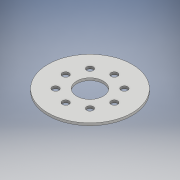
# Autodesk Inventor part: motor_spacer_leg
Saved by Autodesk Inventor 2018 (Build 220112000, 112)
## iProperties
Created: 2018-05-21
Part Number: motor_spacer_leg
Material: Generic
Document SubType Name: Modeling
Designer: bitbots
Density: 1 g/cm^3
Appearance: Default
Author: bitbots
Autodesk Inventor part; units mm, degrees
ref_plane "YZ Plane" through (0, 0, 0) normal (1, 0, 0) x (0, 1, 0)
ref_plane "XZ Plane" through (0, 0, 0) normal (0, 1, 0) x (-1, 0, 0)
ref_plane "XY Plane" through (0, 0, 0) normal (0, 0, 1) x (1, 0, 0)
sketch "Sketch1" plane through (0, 0, 0) normal (0, 0, 1) x (1, 0, 0)
  line L0 (-13, -11) -> (13, -11) construction
  circle A0 centre (0, 0) radius 13.8 construction
  circle A1 centre (0, 0) radius 5 construction
  circle A2 centre (0, -11) radius 1.2813 construction
  circle A3 centre (-7.7782, -7.7782) radius 1.2813 construction
  circle A4 centre (-11, 0) radius 1.2813 construction
  circle A5 centre (-7.7782, 7.7782) radius 1.2813 construction
  circle A6 centre (0, 11) radius 1.2813 construction
  circle A7 centre (7.7782, 7.7782) radius 1.2813 construction
  circle A8 centre (11, 0) radius 1.2813 construction
  circle A9 centre (7.7782, -7.7782) radius 1.2813 construction
  circle A10 centre (0, -8) radius 1.2 construction
  circle A11 centre (-8, 0) radius 1.2 construction
  circle A12 centre (0, 8) radius 1.2 construction
  circle A13 centre (8, 0) radius 1.2 construction
  circle A14 centre (0, -11) radius 1.5
  circle A15 centre (7.7782, -7.7782) radius 1.5
  circle A16 centre (11, 0) radius 1.5
  circle A17 centre (7.7782, 7.7782) radius 1.5
  circle A18 centre (0, 11) radius 1.5
  circle A19 centre (-7.7782, 7.7782) radius 1.5
  circle A20 centre (-11, 0) radius 1.5
  circle A21 centre (-7.7782, -7.7782) radius 1.5
  circle A22 centre (0, 0) radius 6
  circle A23 centre (0, 0) radius 19
  dimension "d0" = 3
  dimension "d3" = 360
  dimension "d5" = 12
  dimension "d6" = 38
  constraints: 10 centre point, 3 coincident, 17 other
  measures "d0" diameter of A14
  measures "d5" diameter of A22
  measures "d6" diameter of A23
extrude "Extrusion1" add sketch "Sketch1" along normal blind 1.1
body "Solid1"
